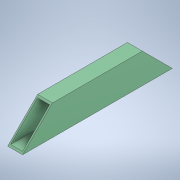
# Autodesk Inventor part: PerfilD1
Saved by Autodesk Inventor 2021 (Build 250183000, 183)
## iProperties
Created: 2021-06-11
Part Number: PerfilD1
Material: Generic
Document SubType Name: Modeling
Designer: lcper
Density: 1 g/cm^3
Appearance: Default
Author: lcper
Autodesk Inventor part; units mm, degrees
ref_plane "YZ Plane" through (0, 0, 0) normal (1, 0, 0) x (0, 1, 0)
ref_plane "XZ Plane" through (0, 0, 0) normal (0, 1, 0) x (-1, 0, 0)
ref_plane "XY Plane" through (0, 0, 0) normal (0, 0, 1) x (1, 0, 0)
sketch "Sketch1" plane through (0, 0, 0) normal (0, 0, 1) x (1, 0, 0)
  line L0 (-9.4777, 15.0257) -> (40.5223, 15.0257)
  line L1 (40.5223, 15.0257) -> (40.5223, -84.9743)
  line L2 (40.5223, -84.9743) -> (-9.4777, -84.9743)
  line L3 (-9.4777, -84.9743) -> (-9.4777, 15.0257)
  line L4 (35.5223, 10.0257) -> (-4.4777, 10.0257)
  line L5 (-4.4777, 10.0257) -> (-4.4777, -79.9743)
  line L6 (-4.4777, -79.9743) -> (35.5223, -79.9743)
  line L7 (35.5223, -79.9743) -> (35.5223, 10.0257)
  point P0 (0, 0)
  point P1 (0, 0)
  dimension "d0" = 50
  dimension "d1" = 100
  dimension "d2" = 5
  dimension "d3" = 90
  dimension "d4" = 5
  dimension "d5" = 40
  constraints: 16 end point, 4 parallel, 2 horizontal, 2 perpendicular
  measures "d0" distance of L1.end L2.end
  measures "d1" distance of L0.end L1.end
  measures "d2" distance between parallel lines of L4 L0
  measures "d3" distance of L6.end L4.start
  measures "d4" distance between parallel lines of L1 L7
  measures "d5" distance of L5.end L6.end
extrude "Extrusion1" add sketch "Sketch1" along normal blind 500
sketch "Sketch2" plane through (40.5223, -84.9743, 0) normal (1, 0, 0) x (0, 0, -1)
  line L0 (-500, 0) -> (-500, 100) projected
  line L1 (-500, 0) -> (-399.1159, 100.8841)
  line L2 (-500, 0) -> (-357.3284, 0) construction
  line L3 (-399.1159, 100.8841) -> (-500, 100.8841)
  line L4 (0, 95) -> (-500, 95) projected
  line L5 (-500, 100.8841) -> (-500, 0)
  line L6 (0, 0) -> (0, 100) projected
  line L7 (0, 0) -> (-100, 100)
  line L8 (0, 0) -> (141.4214, 0) construction
  line L9 (-100, 100) -> (0, 100)
  line L10 (0, 100) -> (0, 0)
  point P0 (0, 84.9743)
  point P1 (-405, 95)
  dimension "d8" = 45
  dimension "d9" = 135
  constraints: 16 end point, 3 perpendicular, 2 equal length, 2 horizontal, 1 parallel, 1 point on line
  measures "d8" angle of L2 L1
  measures "d9" angle of L8 L7
extrude "Extrusion2" cut sketch "Sketch2" against normal blind 50
body "Solid1"
